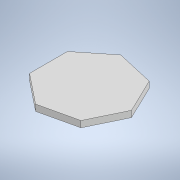
# Autodesk Inventor part: objeto6
Saved by Autodesk Inventor 2022.3 (Build 263350000, 350)
## iProperties
Created: 2023-06-18
Part Number: objeto6
Material: Generic
Document SubType Name: Modeling
Designer: crist
Density: 1 g/cm^3
Appearance: Default
Author: crist
Autodesk Inventor part; units mm, degrees
ref_plane "YZ Plane" through (0, 0, 0) normal (1, 0, 0) x (0, 1, 0)
ref_plane "XZ Plane" through (0, 0, 0) normal (0, 1, 0) x (-1, 0, 0)
ref_plane "XY Plane" through (0, 0, 0) normal (0, 0, 1) x (1, 0, 0)
sketch "Sketch1" plane through (0, 0, 0) normal (0, 1, 0) x (-1, 0, 0)
  circle A0 centre (0, 0) radius 25 construction
  line L0 (25, -12.0394) -> (6.1745, -27.0522)
  line L1 (6.1745, -27.0522) -> (-17.3005, -21.6942)
  line L2 (-17.3005, -21.6942) -> (-27.7479, 0)
  line L3 (-27.7479, 0) -> (-17.3005, 21.6942)
  line L4 (-17.3005, 21.6942) -> (6.1745, 27.0522)
  line L5 (6.1745, 27.0522) -> (25, 12.0394)
  line L6 (25, 12.0394) -> (25, -12.0394)
  point P0 (25, 0)
  dimension "d0" = 50
  constraints: 14 end point, 2 coincident, 1 horizontal alignment, 1 midpoint, 17 other
extrude "Extrusion1" add sketch "Sketch1" along normal blind 4
body "Solid1"
